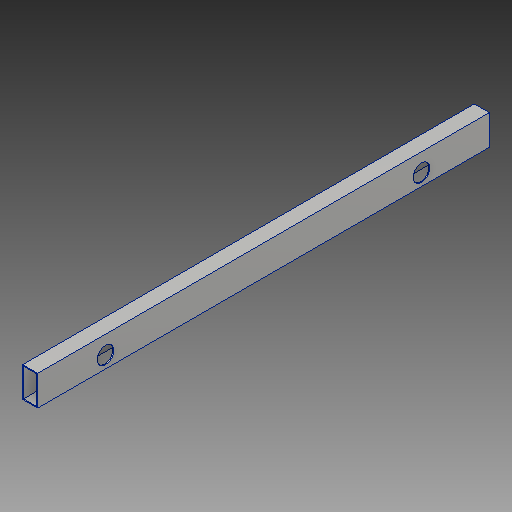
# Autodesk Inventor part: sides
Saved by Autodesk Inventor 2018 (Build 220112000, 112)
## iProperties
Created: 2019-03-28
Part Number: sides
Material: Aluminum 6061
Document SubType Name: Modeling
Designer: corbin
Density: 2.7 g/cm^3
Appearance: Aluminum - Flat
Author: corbin
Autodesk Inventor part; units mm, degrees
ref_plane "YZ Plane" through (0, 0, 0) normal (1, 0, 0) x (0, 1, 0)
ref_plane "XZ Plane" through (0, 0, 0) normal (0, 1, 0) x (-1, 0, 0)
ref_plane "XY Plane" through (0, 0, 0) normal (0, 0, 1) x (1, 0, 0)
sketch "Sketch1" plane through (0, 0, 0) normal (0, 0, 1) x (1, 0, 0)
  line L0 (-12.7, -25.4) -> (12.7, -25.4)
  line L1 (12.7, -25.4) -> (12.7, 25.4)
  line L2 (12.7, 25.4) -> (-12.7, 25.4)
  line L3 (-12.7, 25.4) -> (-12.7, -25.4)
  line L4 (-12.7, -25.4) -> (12.7, 25.4) construction
  line L5 (12.7, -25.4) -> (-12.7, 25.4) construction
  line L6 (-11.1252, 23.8252) -> (11.1252, 23.8252)
  line L7 (11.1252, 23.8252) -> (11.1252, -23.8252)
  line L8 (11.1252, -23.8252) -> (-11.1252, -23.8252)
  line L9 (-11.1252, -23.8252) -> (-11.1252, 23.8252)
  line L10 (-11.1252, 23.8252) -> (11.1252, -23.8252) construction
  line L11 (11.1252, 23.8252) -> (-11.1252, -23.8252) construction
  point P0 (0, 0)
  dimension "d0" = 25.4
  dimension "d1" = 50.8
  dimension "d2" = 22.2504
  dimension "d3" = 47.6504
  constraints: 24 end point, 4 midpoint, 4 parallel, 2 horizontal, 2 perpendicular
  measures "d0" distance of L2.end L1.end
  measures "d1" distance of L1.end L0.end
  measures "d2" distance of L6.start L6.end
  measures "d3" distance of L6.end L7.end
extrude "Extrusion2" add sketch "Sketch1" along normal blind 762
hole "Hole1" at (12.7, -5.08, 114.4016) direction (-1, 0, 0) diameter 28.575 depth 5.08 tip angle 118
hole "Hole2" at (12.7, -5.08, 647.5984) direction (-1, 0, 0) diameter 28.575 depth 5.08 tip angle 118
body "Solid4"
